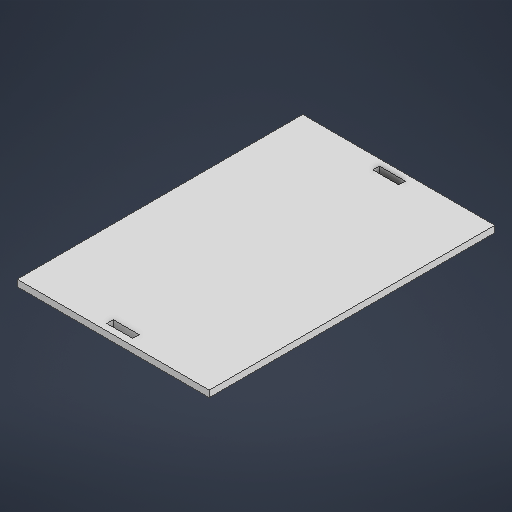
# Autodesk Inventor part: Part1
Saved by Autodesk Inventor 2026 (Build 300175050, 175E)
## iProperties
Created: 2025-06-06
Part Number: Part1
Material: Generic
Document SubType Name: Modeling
Designer: HP
Density: 1 g/cm^3
Appearance: Default
Author: HP
Autodesk Inventor part; units mm, degrees
ref_plane "YZ Plane" through (0, 0, 0) normal (1, 0, 0) x (0, 1, 0)
ref_plane "XZ Plane" through (0, 0, 0) normal (0, 1, 0) x (-1, 0, 0)
ref_plane "XY Plane" through (0, 0, 0) normal (0, 0, 1) x (1, 0, 0)
sketch "Sketch1" plane through (0, 0, 0) normal (0, 1, 0) x (-1, 0, 0)
  line L0 (0, 0) -> (148, 0)
  line L1 (148, 0) -> (148, -220)
  line L2 (148, -220) -> (0, -220)
  line L3 (0, -220) -> (0, 0)
  dimension "d0" = 148
  dimension "d1" = 220
  constraints: 8 end point, 2 parallel, 1 horizontal, 1 perpendicular
  measures "d0" distance of L1.end L2.end
  measures "d1" distance of L0.end L1.end
extrude "Extrusion1" add sketch "Sketch1" along normal blind 5
sketch "Sketch2" plane through (0, 5, 0) normal (0, 1, 0) x (1, 0, 0)
  line L0 (-84, 10) -> (-64, 10)
  line L1 (-64, 10) -> (-64, 5)
  line L2 (-64, 5) -> (-84, 5)
  line L3 (-84, 5) -> (-84, 10)
  line L4 (-148, 0) -> (0, 0) projected
  line L5 (0, 0) -> (0, 220) projected
  line L6 (-84, 215) -> (-64, 215)
  line L7 (-64, 215) -> (-64, 210)
  line L8 (-64, 210) -> (-84, 210)
  line L9 (-84, 210) -> (-84, 215)
  line L10 (0, 220) -> (-148, 220) projected
  point P0 (-64, 7.5)
  point P1 (-64, 212.5)
  point P2 (-74, 220)
  point P3 (-74, 215)
  dimension "d4" = 20
  dimension "d5" = 5
  dimension "d6" = 5
  dimension "d7" = 64
  dimension "d8" = 20
  dimension "d9" = 5
  dimension "d10" = 64
  dimension "d11" = 5
  constraints: 16 end point, 4 midpoint, 4 parallel, 2 horizontal, 2 perpendicular
  measures "d4" distance of L1.end L2.end
  measures "d5" distance of L0.end L1.end
  measures "d6" distance between parallel lines of L4 L2
  measures "d7" distance from line of L5 point (-64, 7.5)
  measures "d8" distance of L7.end L8.end
  measures "d9" distance of L6.end L7.end
  measures "d10" distance from line of L5 point (-64, 212.5)
  measures "d11" distance of point (-74, 220) point (-74, 215)
extrude "Extrusion2" cut sketch "Sketch2" against normal through all
body "Solid1"
